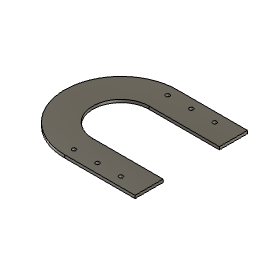
Cover (Autodesk Fusion 360 design; units mm, degrees)
Autodesk Fusion 360 part; units mm, degrees
sketch "草图1" plane through (0, 0, 0) normal (0, 0, 1) x (1, 0, 0)
  line L0 (0, 60) -> (75, 60)
  line L1 (75, 60) -> (75, 30)
  line L2 (75, 30) -> (0, 30)
  line L3 (0, -60) -> (75, -60)
  line L4 (75, -60) -> (75, -30)
  line L5 (75, -30) -> (0, -30)
  arc A0 (0, 60) -> (0, -60) centre (0, 0) ccw
  arc A1 (0, 30) -> (0, -30) centre (0, 0) ccw
  circle A2 centre (0, 50) radius 2.1
  circle A3 centre (25, 50) radius 2.1
  circle A4 centre (50, 50) radius 2.1
  circle A5 centre (0, -50) radius 2.1
  circle A6 centre (25, -50) radius 2.1
  circle A7 centre (50, -50) radius 2.1
  dimension "d1" = 4.2
  dimension "d2" = 4.2
  dimension "d3" = 4.2
  dimension "d4" = 4.2
  dimension "d5" = 4.2
  dimension "d6" = 4.2
  constraint coincident A0.centre A1.centre
  constraint concentric A0 A1
  constraint horizontal L0
  constraint vertical L1
  constraint horizontal L2
  constraint horizontal L3
  constraint vertical L4
  constraint horizontal L5
  measures "d1" diameter of A2
  measures "d2" diameter of A3
  measures "d3" diameter of A4
  measures "d4" diameter of A5
  measures "d5" diameter of A6
  measures "d6" diameter of A7
extrude "拉伸1" add sketch "草图1" along normal blind 3
sketch "草图2" plane through (0, 0, 0) normal (0, 1, 0) x (1, 0, 0)
sketch "草图3" plane through (0, 0, 0) normal (0, 0, 1) x (1, 0, 0)
